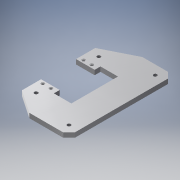
# Autodesk Inventor part: Support_Roue
Saved by Autodesk Inventor 2016 (Build 200138000, 138)
## iProperties
Created: 2015-09-29
Part Number: Support_Roue
Material: Générique
Document SubType Name: Modeling
Designer: Logan
Density: 1 g/cm^3
Appearance: Par défaut
Author: Logan
Autodesk Inventor part; units mm, degrees
ref_plane "YZ Plane" through (0, 0, 0) normal (1, 0, 0) x (0, 1, 0)
ref_plane "XZ Plane" through (0, 0, 0) normal (0, 1, 0) x (-1, 0, 0)
ref_plane "XY Plane" through (0, 0, 0) normal (0, 0, 1) x (1, 0, 0)
sketch "Esquisse1" plane through (0, 0, 0) normal (0, 0, 1) x (1, 0, 0)
  line L0 (-44, 90) -> (-88, 90)
  line L1 (-102, -90) -> (-44, -90)
  line L2 (-34, -80) -> (-34, 80)
  line L3 (-88, 90) -> (-142, 63)
  line L4 (-102, -90) -> (-142, -63)
  line L5 (-44, 90) -> (-34, 80)
  line L6 (-44, -90) -> (-34, -80)
  line L7 (-80, 40) -> (-110, 40)
  line L8 (-110, -40) -> (-80, -40)
  line L9 (-80, -40) -> (-80, 40)
  line L10 (-142, 30) -> (-110, 30)
  line L11 (-110, -30) -> (-142, -30)
  line L12 (-142, 63) -> (-142, 30)
  line L13 (-142, -30) -> (-142, -63)
  line L14 (-110, 40) -> (-110, 30)
  line L15 (-110, -30) -> (-110, -40)
  line L16 (346.6566, 90) -> (-88, 90)
  point P0 (0, 0)
  point P1 (-34, 90)
  point P2 (-142, -90)
  point P3 (-142, 90)
  point P4 (-34, -90)
  dimension "d10" = 180
  dimension "d15" = 54
  dimension "d16" = 27
  dimension "d17" = 40
  dimension "d18" = 27
  dimension "d19" = 10
  dimension "d20" = 10
  dimension "d21" = 10
  dimension "d22" = 10
  dimension "d23" = 80
  dimension "d25" = 40
  dimension "d26" = 46
  dimension "d28" = 60
  dimension "d29" = 30
  dimension "d53" = 108
  dimension "d55" = 90
  dimension "d56" = 80
  dimension "d75" = 108
  dimension "d76" = 108
  dimension "d77" = 76
  dimension "d79" = 32
  dimension "d97" = 90
  constraints: 34 end point, 7 parallel, 7 point on line, 4 horizontal, 4 perpendicular, 2 collinear
  measures "d10" distance between parallel lines of L1 L0
  measures "d15" distance of L0.end point (-142, 90)
  measures "d16" distance of L3.end point (-142, 90)
  measures "d17" distance of L1.start point (-142, -90)
  measures "d18" distance of L4.end point (-142, -90)
  measures "d19" distance of L0.start point (-34, 90)
  measures "d20" distance of L2.end point (-34, 90)
  measures "d21" distance of L1.end point (-34, -90)
  measures "d22" distance of L2.start point (-34, -90)
  measures "d23" distance between parallel lines of L8 L7
  measures "d25" distance from line of point (0, 0) L8
  measures "d26" distance between parallel lines of L2 L9
  measures "d28" distance between parallel lines of L11 L10
  measures "d29" distance from line of point (0, 0) L10
  measures "d53" distance between parallel lines of L2 L12
  measures "d55" distance from line of point (0, 0) L1
  measures "d56" distance from line of point (0, 0) L9
  measures "d75" distance from line of L2 point (-142, -90)
  measures "d76" distance from line of L2 point (-142, 90)
  measures "d77" distance between parallel lines of L2 L15
  measures "d79" distance of L10.start L10.end
  measures "d97" distance from line of point (0, 0) L16
extrude "Plaque" add sketch "Esquisse1" along normal blind 8
sketch "Esquisse2" plane through (0, 0, 8) normal (0, 0, 1) x (1, 0, 0)
  line L0 (-80, 40) -> (-80, -40) projected
  line L1 (-80, -40) -> (-110, -40) projected
  line L2 (-110, 30) -> (-110, 40) projected
  line L3 (-110, 40) -> (-80, 40) projected
  line L4 (-88, 90) -> (-142, 63) projected
  line L5 (-142, 63) -> (-142, 30) projected
  line L6 (-142, 30) -> (-110, 30) projected
  line L7 (-110, -30) -> (-142, -30) projected
  line L8 (-142, -30) -> (-142, -63) projected
  line L9 (-142, -63) -> (-102, -90) projected
  line L10 (-102, -90) -> (-44, -90) projected
  line L11 (-44, -90) -> (-34, -80) projected
  line L12 (-34, -80) -> (-34, 80) projected
  line L13 (-34, 80) -> (-44, 90) projected
  line L14 (-44, 90) -> (-88, 90) projected
  circle A0 centre (-120, -35) radius 2
  circle A1 centre (-134, -35) radius 2
  circle A2 centre (-120, 35) radius 2
  circle A3 centre (-134, 35) radius 2
  line L15 (-110, -40) -> (-110, -30) projected
  dimension "d33" = 4
  dimension "d34" = 4
  dimension "d35" = 4
  dimension "d36" = 4
  dimension "d38" = 5
  dimension "d39" = 5
  dimension "d40" = 5
  dimension "d41" = 5
  dimension "d42" = 14
  dimension "d43" = 14
  dimension "d80" = 10
  dimension "d81" = 10
  dimension "d82" = 8
  constraints: 4 centre point
  measures "d33" diameter of A0
  measures "d34" diameter of A1
  measures "d35" diameter of A2
  measures "d36" diameter of A3
  measures "d38" distance from line of A1.centre L7
  measures "d39" distance from line of L7 A0.centre
  measures "d40" distance from line of L6 A2.centre
  measures "d41" distance from line of L6 A3.centre
  measures "d42" distance of A0.centre A1.centre
  measures "d43" distance of A2.centre A3.centre
  measures "d80" distance from line of L2 A2.centre
  measures "d81" distance from line of L15 A0.centre
  measures "d82" distance from line of L5 A3.centre
hole "Fixation_Encodeur" at (-134, 35, 8) at (-120, 35, 8) at (-134, -35, 8) at (-120, -35, 8) direction (0, 0, -1) diameter 4 end through all
sketch "Esquisse3" plane through (0, 0, 8) normal (0, 0, 1) x (1, 0, 0)
  line L0 (-80, 40) -> (-80, -40) projected
  line L1 (-80, -40) -> (-110, -40) projected
  line L2 (-110, 30) -> (-110, 40) projected
  line L3 (-110, 40) -> (-80, 40) projected
  line L4 (-88, 90) -> (-142, 63) projected
  line L5 (-142, 63) -> (-142, 30) projected
  line L6 (-142, 30) -> (-110, 30) projected
  line L7 (-110, -30) -> (-142, -30) projected
  line L8 (-142, -30) -> (-142, -63) projected
  line L9 (-142, -63) -> (-102, -90) projected
  line L10 (-102, -90) -> (-44, -90) projected
  line L11 (-44, -90) -> (-34, -80) projected
  line L12 (-34, -80) -> (-34, 80) projected
  line L13 (-34, 80) -> (-44, 90) projected
  line L14 (-44, 90) -> (-88, 90) projected
  line L15 (-110, -40) -> (-110, -30) projected
  circle A0 centre (-134, -35) radius 2 projected
  circle A1 centre (-134, 35) radius 2 projected
  circle A2 centre (-120, 35) radius 2 projected
  circle A3 centre (-120, -35) radius 2 projected
  line L16 (-88, 90) -> (-142, 63) projected
  line L17 (-142, 63) -> (-142, 30) projected
  line L18 (-142, 30) -> (-110, 30) projected
  line L19 (-110, 30) -> (-110, 40) projected
  line L20 (-110, 40) -> (-80, 40) projected
  line L21 (-80, 40) -> (-80, -40) projected
  line L22 (-80, -40) -> (-110, -40) projected
  line L23 (-110, -40) -> (-110, -30) projected
  line L24 (-110, -30) -> (-142, -30) projected
  line L25 (-142, -30) -> (-142, -63) projected
  line L26 (-142, -63) -> (-102, -90) projected
  line L27 (-102, -90) -> (-44, -90) projected
  line L28 (-44, -90) -> (-34, -80) projected
  line L29 (-34, -80) -> (-34, 80) projected
  line L30 (-34, 80) -> (-44, 90) projected
  line L31 (-44, 90) -> (-88, 90) projected
  line L32 (-126, 53.1115) -> (-84.2229, 74)
  line L33 (-84.2229, 74) -> (-50, 74)
  line L34 (-50, 74) -> (-50, -74)
  line L35 (-50, -74) -> (-97.1054, -74)
  line L36 (-97.1054, -74) -> (-126, -54.4961)
  dimension "d103" = 16
  constraints: 10 end point
  measures "d103" distance between parallel lines of L4 L32
hole "Fixation_Plaque" at (-126, 53.1115, 8) at (-50, 74, 8) at (-50, -74, 8) at (-126, -54.4961, 8) direction (0, 0, -1) diameter 6 end through all
chamfer "Passage_Vis" distance 1 angle 45 8 edges at (-134, 37, 8) (-120, 37, 8) (-120, -33, 8) (-134, -33, 8) (-134, 37, 0) (-120, 37, 0) (-120, -33, 0) (-134, -33, 0)
equation "\"d20\" = d19"
equation "\"d21\" = d19"
equation "\"d22\" = d21"
